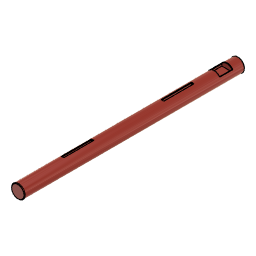
prototipo 1 (Autodesk Fusion 360 design; units mm, degrees)
Autodesk Fusion 360 part; units mm, degrees
sketch "Boceto1" plane through (0, 0, 0) normal (0, 1, 0) x (1, 0, 0)
  circle A0 centre (0, 0) radius 37
  dimension "d1" = 74
  constraint coincident A0.centre origin
  measures "d1" diameter of A0
extrude "Extruir1" add sketch "Boceto1" along normal blind 1200
ref_plane "PlanoDeObra1" through (0, 0, 39.368) normal (0, 0, 1) x (1, 0, 0)
sketch "Boceto2" plane through (0, 0, 39.368) normal (0, 0, 1) x (1, 0, 0)
  line L0 (0, 0) -> (0, 250) construction
  line L1 (0, 250) -> (0, 410.6)
  line L2 (0, 410.6) -> (-10, 410.6)
  line L3 (-10, 410.6) -> (-10, 250)
  line L4 (-10, 250) -> (0, 250)
  line L5 (0.0066, 950.0297) -> (-4.9934, 950.0297)
  line L6 (-4.9934, 950.0297) -> (-4.9934, 789.4297)
  line L7 (0.0066, 950.0297) -> (5.0066, 950.0297)
  line L8 (5.0066, 950.0297) -> (5.0066, 789.4297)
  line L9 (5.0066, 789.4297) -> (-4.9934, 789.4297)
  line L10 (27.0066, 1138.525) -> (-26.9934, 1138.525)
  line L11 (-26.9934, 1138.525) -> (-26.9934, 1070.525)
  line L12 (-26.9934, 1070.525) -> (27.0066, 1070.525)
  line L13 (27.0066, 1070.525) -> (27.0066, 1138.525)
  line L14 (27.0066, 1138.525) -> (-26.9934, 1070.525) construction
  line L15 (-26.9934, 1138.525) -> (27.0066, 1070.525) construction
  point P0 (0.0066, 1104.525)
  dimension "d5" = 250
  dimension "d6" = 160.6
  dimension "d7" = 10
  dimension "d8" = 160.6
  dimension "d18" = 5
  dimension "d19" = 160.6
  dimension "d20" = 5
  dimension "d21" = 160.6
  dimension "d26" = 54
  dimension "d27" = 68
  constraint coincident L0.start origin
  constraint vertical L0
  constraint parallel L0 L1
  constraint perpendicular L1 L2
  constraint perpendicular L2 L3
  constraint perpendicular L5 L6
  constraint perpendicular L7 L8
  constraint horizontal L10
  constraint perpendicular L10 L11
  constraint parallel L10 L12
  constraint parallel L11 L13
  constraint coincident L14 P0
  constraint coincident L15 P0
  measures "d5" distance of L0.start L0.end
  measures "d6" distance of L0.end L1.end
  measures "d7" distance of L1.end L2.end
  measures "d8" distance of L2.end L3.end
  measures "d18" distance of L5.start L5.end
  measures "d19" distance of L5.end L6.end
  measures "d20" distance of L5.start L7.end
  measures "d21" distance of L7.end L8.end
  measures "d26" distance of L11.end L12.end
  measures "d27" distance of L10.end L11.end
extrude "Extruir2" cut sketch "Boceto2" against normal blind 40 contours L1 L2 L3 L4
fillet "Empalme1" radius 2 4 edges at (-10, 330.3, 35.623) (-5.0472, 410.6, 36.6541) (0, 330.3, 37) (-5.0472, 250, 36.6541)
extrude "Extruir3" cut sketch "Boceto2" against normal blind 40 contours L5 L6 L7 L8 L9
fillet "Empalme2" radius 2 4 edges at (-4.9934, 869.7297, 36.6615) (0.0067, 950.0297, 37) (5.0066, 869.7297, 36.6597) (0.0067, 789.4297, 37)
extrude "Extruir4" cut sketch "Boceto2" against normal blind 20 contours L10 L11 L12 L13
fillet "Empalme3" radius 2 4 edges at (-26.9934, 1104.525, 25.3053) (0.0097, 1138.525, 37) (27.0066, 1104.525, 25.2911) (0.0097, 1070.525, 37)
extrude "Extruir5" cut 1 faces at (-8.9934, 1093.1916, 19.368) along direction (0, 0, -1) blind 10
fillet "Empalme4" radius 3 1 edges at (-34.4961, 0, 13.3798)
fillet "Empalme5" radius 3 1 edges at (-34.4961, 1200, 13.3798)
